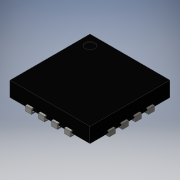
# Autodesk Inventor part: MLPQ
Saved by Autodesk Inventor 2016 (Build 200138000, 138)
## iProperties
Created: 2016-07-01
Part Number: MLPQ
Material: Generic
Document SubType Name: Modeling
Designer: Jonathan
Density: 1 g/cm^3
Appearance: Default
Author: Jonathan
Autodesk Inventor part; units mm, degrees
ref_plane "YZ Plane" through (0, 0, 0) normal (1, 0, 0) x (0, 1, 0)
ref_plane "XZ Plane" through (0, 0, 0) normal (0, 1, 0) x (-1, 0, 0)
ref_plane "XY Plane" through (0, 0, 0) normal (0, 0, 1) x (1, 0, 0)
sketch "Sketch1" plane through (0, 0, 0) normal (0, 1, 0) x (-1, 0, 0)
  line L0 (2, 2) -> (-2, 2)
  line L1 (-2, 2) -> (-2, -2)
  line L2 (-2, -2) -> (2, -2)
  line L3 (2, -2) -> (2, 2)
  point P0 (0, 0)
  point P1 (0, -2)
  point P2 (2, 0)
  dimension "d0" = 4
  dimension "d1" = 4
  constraints: 8 end point, 2 midpoint, 2 parallel, 1 horizontal, 1 horizontal alignment, 1 perpendicular, 1 vertical alignment
  measures "d0" distance of L2.end L0.start
  measures "d1" distance of L1.end L2.end
extrude "Extrusion1" add sketch "Sketch1" along normal blind 0.75
sketch "Sketch2" plane through (2, 0, 2) normal (1, 0, 0) x (0, 0, -1)
  line L0 (0.875, 0.15) -> (1.175, 0.15)
  line L1 (1.175, 0.15) -> (1.175, 0.1)
  line L2 (1.175, 0.1) -> (0.875, 0.1)
  line L3 (0.875, 0.1) -> (0.875, 0.15)
  line L4 (0, 0) -> (4, 0) projected
  point P0 (2, 0)
  point P1 (1.025, 0.15)
  dimension "d4" = 0.975
  dimension "d5" = 0.3
  dimension "d6" = 0.05
  dimension "d10" = 0.1
  constraints: 8 end point, 2 parallel, 1 horizontal, 1 midpoint, 1 perpendicular
  measures "d4" horizontal distance of point (2, 0) point (1.025, 0.15)
  measures "d5" distance of L0.start L0.end
  measures "d6" distance of L2.end L0.start
  measures "d10" distance between parallel lines of L4 L2
extrude "Extrusion2" add sketch "Sketch2" along normal blind 0.1 separate body
sketch "Sketch4" plane through (2, 0.1, 0.825) normal (0, -1, 0) x (1, 0, 0)
  line L0 (0.1, 0) -> (0.1, 0.3) projected
  line L1 (0, 0) -> (0.1, 0) projected
  line L2 (0.1, 0.3) -> (0.05, 0.3)
  line L3 (0.05, 0.3) -> (0.05, 0)
  line L4 (0.05, 0) -> (0.1, 0)
  line L5 (0.1, 0) -> (0.1, 0.3)
  point P0 (-2, -0.825)
  dimension "d11" = 0.05
  constraints: 8 end point, 2 parallel, 1 horizontal, 1 midpoint, 1 perpendicular
  measures "d11" distance between parallel lines of L3 L0
extrude "Extrusion3" add sketch "Sketch4" along normal blind 0.2 bodies 2
sketch "Sketch7" plane through (2, -0.1, 0.825) normal (0, -1, 0) x (1, 0, 0)
  line L0 (0, 0.3) -> (0.1, 0.3) projected
  line L1 (0.05, 0.3) -> (-0.25, 0.3)
  line L2 (0.05, 0.3) -> (0.05, 0) projected
  line L3 (0.05, 0) -> (-0.25, 0)
  arc A0 (-0.25, 0.3) -> (-0.25, 0) centre (-0.25, 0.15) ccw
  line L4 (0.05, 0.3) -> (0.05, 0)
  line L5 (-0.4, 0.4) -> (-0.4, -0.1) construction
  line L6 (0, 1.175) -> (0, -2.825) projected
  point P0 (-2, -0.825)
  point P1 (-0.4, 0.15)
  dimension "d38" = 0.5
  dimension "d39" = 0.4
  constraints: 8 end point, 3 point on circle, 2 horizontal, 2 midpoint, 2 tangent, 1 centre point, 1 perpendicular, 1 vertical
  measures "d38" distance of L5.start L5.end
  measures "d39" distance between parallel lines of L6 L5
extrude "Extrusion5" add sketch "Sketch7" against normal blind 0.05 bodies 2
fillet "Fillet1" radius 0.01 4 edges at (2.1, -0.1, 0.975) (2.1, 0.15, 0.975) (2.05, -0.05, 0.975) (2.05, 0.1, 0.975)
sketch "Sketch8" plane through (0, 0.75, 0) normal (0, 1, 0) x (1, 0, 0)
  circle A0 centre (-1.5, 1.5) radius 0.25
  line L0 (2, 2) -> (-2, 2) projected
  line L1 (-2, 2) -> (-2, -2) projected
  point P0 (0, 0)
  dimension "d29" = 0.5
  dimension "d30" = 0.5
  dimension "d31" = 0.5
  constraints: 1 centre point
  measures "d29" diameter of A0
  measures "d30" distance from line of L0 A0.centre
  measures "d31" distance from line of L1 A0.centre
extrude "Extrusion6" cut sketch "Sketch8" against normal blind 0.05 bodies 1
sketch "Sketch9" plane through (0, 0, 0) normal (0, -1, 0) x (1, 0, 0)
  line L0 (-1.35, 1.35) -> (1.35, 1.35)
  line L1 (1.35, 1.35) -> (1.35, -1.35)
  line L2 (1.35, -1.35) -> (-0.9964, -1.35)
  line L3 (-1.35, -0.9964) -> (-1.35, 1.35)
  line L4 (-1.35, -0.9964) -> (-0.9964, -1.35)
  point P0 (0, 0)
  point P1 (0, 1.35)
  point P2 (1.35, 0)
  dimension "d34" = 2.7
  dimension "d35" = 0.5
  constraints: 10 end point, 3 perpendicular, 2 midpoint, 2 parallel, 1 horizontal, 1 horizontal alignment, 1 vertical alignment
  measures "d34" distance of L0.end L1.end
  measures "d35" distance of L3.start L2.end
extrude "Extrusion7" add sketch "Sketch9" along normal blind 0.05 bodies 2
pattern_linear "Rectangular Pattern2" count 4 spacing 0.65 along (0, 0, -1) of "Extrusion5", "Extrusion3", "Extrusion2" bodies 2
pattern_circular "Circular Pattern2" count 4 over 360 about axis through (0, -10, 0) along (0, 1, 0) of "Extrusion5", "Extrusion3", "Extrusion2", "Rectangular Pattern2" bodies 2
body "Solid1"
body "Solid2"
